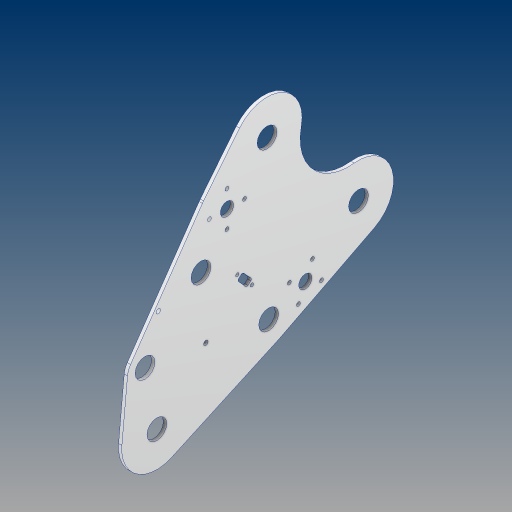
# Autodesk Inventor part: SHOT_1_001_ShooterPlate
Saved by Autodesk Inventor 2024.3 (Build 283343000, 343)
## iProperties
Created: 2024-08-07
Part Number: SHOT_1_001_ShooterPlate
Material: Aluminum 6061
Document SubType Name: Modeling
Designer: Kenji
Density: 2.7 g/cm^3
Appearance: Aluminum - Flat
Mass: 320.131 g
Surface Area: 825.953 cm^2
Volume: 118.567 cm^3
Author: Kenji
Autodesk Inventor part; units mm, degrees
ref_plane "YZ Plane" through (0, 0, 0) normal (1, 0, 0) x (0, 1, 0)
ref_plane "XZ Plane" through (0, 0, 0) normal (0, 1, 0) x (-1, 0, 0)
ref_plane "XY Plane" through (0, 0, 0) normal (0, 0, 1) x (1, 0, 0)
sketch "Sketch1" plane through (0, 0, 0) normal (1, 0, 0) x (0, 1, 0)
  line L0 (0, 0) -> (355.6, 0) construction
  line L1 (0, -355.6) -> (0, 0) construction
  line L2 (0, -292.1) -> (279.4, -292.1) construction
  circle A0 centre (336.7111, -261.0807) radius 50.8 construction
  circle A1 centre (191.0749, -393.5194) radius 50.8 construction
  circle A2 centre (263.893, -327.3) radius 50.8 construction
  circle A3 centre (191.0749, -393.5194) radius 47.625 construction
  circle A4 centre (336.7111, -261.0807) radius 47.625 construction
  line L3 (336.7111, -261.0807) -> (191.0749, -393.5194) construction
  circle A5 centre (336.7111, -261.0807) radius 14.2875
  circle A6 centre (191.0749, -393.5194) radius 14.2875
  circle A7 centre (215.3861, -165.4189) radius 25.4 construction
  circle A8 centre (107.6199, -263.4194) radius 25.4 construction
  circle A9 centre (107.6199, -263.4194) radius 22.225 construction
  circle A10 centre (215.3861, -165.4189) radius 22.225 construction
  circle A11 centre (215.3861, -165.4189) radius 14.2875
  circle A12 centre (107.6199, -263.4194) radius 14.2875
  line L4 (301.4765, -293.1223) -> (198.9433, -180.3717) construction
  line L5 (226.3095, -361.4778) -> (123.7762, -248.7272) construction
  circle A13 centre (161.3598, -214.5495) radius 50.8 construction
  line L6 (215.3861, -165.4189) -> (107.6199, -263.4194) construction
  circle A14 centre (50.8, -101.6) radius 50.8 construction
  circle A15 centre (25.4, -170.0653) radius 25.4 construction
  circle A16 centre (25.4, -170.0653) radius 22.225 construction
  circle A17 centre (25.4, -170.0653) radius 14.2875 construction
  circle A18 centre (136.3874, -84.4507) radius 25.4 construction
  circle A19 centre (136.3874, -84.4507) radius 22.225 construction
  circle A20 centre (136.3874, -84.4507) radius 14.2875
  circle A21 centre (50.8, -101.6) radius 14.2875
  circle A22 centre (41.2055, -25.7462) radius 25.4 construction
  circle A23 centre (41.2055, -25.7462) radius 22.225 construction
  circle A24 centre (41.2055, -25.7462) radius 14.2875 construction
  circle A25 centre (-111.1945, -98.7712) radius 50.8 construction
  circle A26 centre (41.2055, -98.7712) radius 50.8 construction
  line L7 (-111.1945, -47.9712) -> (41.2055, -47.9712) construction
  line L8 (-111.1945, -149.5712) -> (41.2055, -149.5712) construction
  circle A27 centre (276.2209, -203.0571) radius 30 construction
  circle A28 centre (276.2209, -203.0571) radius 25.4 construction
  circle A29 centre (301.6209, -203.0571) radius 2.794
  circle A30 centre (294.1814, -185.0966) radius 2.794
  circle A31 centre (276.2209, -177.6571) radius 2.794
  circle A32 centre (258.2604, -185.0966) radius 2.794
  circle A33 centre (250.8209, -203.0571) radius 2.794
  circle A34 centre (258.2604, -221.0176) radius 2.794
  circle A35 centre (276.2209, -228.4571) radius 2.794
  circle A36 centre (294.1814, -221.0176) radius 2.794
  circle A37 centre (276.2209, -203.0571) radius 9.652
  line L9 (250.7089, -187.273) -> (236.9862, -178.7828) construction
  circle A38 centre (276.2209, -203.0571) radius 9.5504 construction
  circle A39 centre (336.7111, -261.0807) radius 9.5504 construction
  circle A40 centre (336.7111, -261.0807) radius 14.3256 construction
  circle A41 centre (215.3861, -165.4189) radius 14.3256 construction
  circle A42 centre (136.3874, -84.4507) radius 14.3256 construction
  circle A43 centre (215.3861, -165.4189) radius 14.3256 construction
  circle A44 centre (123.5241, -172.549) radius 6.35 construction
  circle A45 centre (123.5241, -172.549) radius 3.2512
  line L10 (122.4294, -178.8039) -> (111.9989, -238.3998) construction
  arc A46 (325.875, -310.7115) -> (241.5089, -387.4324) centre (310.9542, -379.0508) ccw
  arc A47 (325.875, -310.7115) -> (368.3984, -221.3748) centre (336.7111, -261.0807) ccw
  arc A48 (145.82, -416.5983) -> (241.5089, -387.4324) centre (191.0749, -393.5194) ccw
  line L11 (138.8602, -59.1713) -> (55.7455, -51.0413)
  arc A49 (150.8617, -63.5783) -> (138.8602, -59.1713) centre (136.3874, -84.4507) ccw
  arc A50 (55.7455, -51.0413) -> (4.5541, -122.6227) centre (50.8, -101.6) ccw
  circle A51 centre (197.6195, -103.7307) radius 6.35 construction
  circle A52 centre (197.6195, -103.7307) radius 3.2512
  line L12 (161.503, -214.4192) -> (263.893, -327.3) construction
  circle A53 centre (128.5074, -316.6157) radius 30 construction
  circle A54 centre (128.5074, -316.6157) radius 25.4 construction
  circle A55 centre (152.1501, -307.3324) radius 2.794 construction
  line L13 (191.5627, -101.8236) -> (160.6148, -92.0791) construction
  line L14 (199.3769, -109.8327) -> (208.3565, -141.0111) construction
  line L15 (116.9032, -287.0622) -> (117.5428, -288.6911) construction
  circle A56 centre (128.5074, -316.6157) radius 22.86 construction
  circle A57 centre (107.6199, -263.4194) radius 34.29 construction
  circle A58 centre (138.661, -293.3334) radius 2.794
  circle A59 centre (119.224, -292.9729) radius 2.794 construction
  circle A60 centre (105.2251, -306.462) radius 2.794
  circle A61 centre (104.8646, -325.899) radius 2.794 construction
  circle A62 centre (118.3537, -339.8979) radius 2.794
  circle A63 centre (137.7907, -340.2584) radius 2.794 construction
  circle A64 centre (151.7896, -326.7693) radius 2.794
  line L16 (176.8412, -219.7225) -> (165.2898, -230.2004)
  line L17 (165.1271, -233.5371) -> (168.7791, -237.5632)
  line L18 (172.1157, -237.7258) -> (183.6672, -227.2479)
  line L19 (183.8298, -223.9112) -> (180.1779, -219.8851)
  arc A65 (183.6672, -227.2479) -> (183.8298, -223.9112) centre (182.0802, -225.4982) ccw
  arc A66 (180.1779, -219.8851) -> (176.8412, -219.7225) centre (178.4283, -221.4722) ccw
  arc A67 (168.7791, -237.5632) -> (172.1157, -237.7258) centre (170.5287, -235.9761) ccw
  arc A68 (165.2898, -230.2004) -> (165.1271, -233.5371) centre (166.8768, -231.9501) ccw
  line L20 (186.1428, -218.1438) -> (162.8049, -239.3128) construction
  circle A69 centre (186.1428, -218.1438) radius 2.3876
  circle A70 centre (162.8049, -239.3128) radius 2.3812
  circle A71 centre (128.5074, -316.6157) radius 9.5504
  circle A72 centre (276.2209, -203.0571) radius 30.48 construction
  circle A73 centre (336.7111, -261.0807) radius 41.91 construction
  circle A74 centre (276.2209, -203.0571) radius 41.91 construction
  circle A75 centre (128.5074, -316.6157) radius 19.1008 construction
  circle A76 centre (215.3861, -165.4189) radius 19.1008 construction
  circle A77 centre (136.3874, -84.4507) radius 19.1008 construction
  circle A78 centre (276.2209, -203.0571) radius 19.1008 construction
  circle A79 centre (191.0749, -393.5194) radius 19.1008 construction
  line L21 (4.5541, -122.6227) -> (75.2478, -278.1353)
  line L22 (75.9415, -279.5746) -> (145.82, -416.5983)
  arc A80 (75.2478, -278.1353) -> (75.9415, -279.5746) centre (107.6199, -263.4194) ccw
  circle A81 centre (276.2209, -203.0571) radius 43.18 construction
  line L23 (303.1551, -169.3072) -> (368.3984, -221.3748)
  line L24 (150.8617, -63.5783) -> (300.8271, -167.5741)
  arc A82 (303.1551, -169.3072) -> (300.8271, -167.5741) centre (276.2209, -203.0571) ccw
  circle A83 centre (107.6199, -263.4194) radius 35.56 construction
  point P0 (33.8339, -53.7169)
  point P1 (178.5909, -218.1355)
  point P2 (163.5401, -231.7874)
  point P3 (170.3661, -239.3128)
  point P4 (171.0655, -224.9614)
  point P5 (182.0039, -221.8981)
  point P6 (182.0039, -221.8981)
  dimension "d44" = 101.6
  dimension "d81" = 60
  dimension "d82" = 50.8
  dimension "d102" = 12.7
  dimension "d268" = 60
  dimension "d269" = 50.8
  dimension "d13" = 355.6
  dimension "d14" = 355.6
  dimension "d15" = 292.1
  dimension "d29" = 101.6
  dimension "d31" = 3.175
  dimension "d36" = 28.575
  dimension "d38" = 50.8
  dimension "d39" = 3.175
  dimension "d41" = 28.575
  dimension "d42" = 152.4
  dimension "d43" = 152.4
  dimension "d46" = 279.4
  dimension "d47" = 101.6
  dimension "d50" = 101.6
  dimension "d51" = 145.6628
  dimension "d60" = 28.575
  dimension "d61" = 113.1223
  dimension "d77" = 101.6
  dimension "d78" = 101.6
  dimension "d79" = 152.4
  dimension "d80" = 41.2055
  dimension "d83" = 5.588
  dimension "d86" = 360
  dimension "d88" = 19.304
  dimension "d91" = 19.1008
  dimension "d92" = 19.1008
  dimension "d93" = 28.6512
  dimension "d94" = 28.6512
  dimension "d95" = 28.6512
  dimension "d96" = 28.6512
  dimension "d103" = 6.5024
  dimension "d108" = 12.7
  dimension "d109" = 6.5024
  dimension "d114" = 101.6
  dimension "d116" = 87.2886
  dimension "d117" = 158.0611
  dimension "d119" = 323.8734
  dimension "d121" = 42.21
  dimension "d270" = 5.588
  dimension "d279" = 45.72
  dimension "d280" = 68.58
  dimension "d283" = 360
  dimension "d285" = 20.32
  dimension "d286" = 10.16
  dimension "d287" = 10.16
  dimension "d288" = 2.3622
  dimension "d289" = 2.3622
  dimension "d291" = 5.08
  dimension "d292" = 4.7752
  dimension "d293" = 4.7625
  dimension "d294" = 5.6005
  dimension "d295" = 5.588
  dimension "d296" = 19.1008
  dimension "d297" = 60.96
  dimension "d300" = 83.82
  dimension "d301" = 83.82
  dimension "d302" = 38.2016
  dimension "d303" = 38.2016
  dimension "d304" = 38.2016
  dimension "d305" = 38.2016
  dimension "d306" = 38.2016
  dimension "d309" = 1.27
  dimension "d312" = 1.27
  dimension "d314" = 208.6282
  constraints: 76 centre point, 50 end point, 46 point on circle, 37 tangent, 32 coincident, 22 point on line, 18 equal radius, 6 midpoint, 5 concentric, 5 perpendicular, 3 horizontal, 2 horizontal alignment, 2 parallel, 1 equal length, 1 vertical alignment, 67 other
  measures "d13" distance of L1.start L0.start
  measures "d14" distance of L0.start L0.end
  measures "d15" distance between parallel lines of L0 L2
  measures "d29" diameter of A1
  measures "d31" radial gap between concentric circles of A1 A3
  measures "d36" diameter of A5
  measures "d38" diameter of A8
  measures "d39" radial gap between concentric circles of A8 A9
  measures "d41" diameter of A12
  measures "d42" distance of L4.start L4.end
  measures "d43" distance of L5.start L5.end
  measures "d46" distance of L2.start L2.end
  measures "d47" diameter of A14
  measures "d50" distance from line of L0 A14.centre
  measures "d51" distance of L6.start L6.end
  measures "d60" diameter of A21
  measures "d61" distance of A19.centre A7.centre
  measures "d77" diameter of A25
  measures "d78" diameter of A26
  measures "d79" distance of L8.start L8.end
  measures "d80" distance from line of L1 A22.centre
  measures "d83" diameter of A29
  measures "d88" diameter of A37
  measures "d91" diameter of A38
  measures "d92" diameter of A39
  measures "d93" diameter of A40
  measures "d94" diameter of A41
  measures "d95" diameter of A42
  measures "d96" diameter of A43
  measures "d103" diameter of A45
  measures "d108" diameter of A51
  measures "d109" diameter of A52
  measures "d114" distance of point (123.524, -172.549) A14.centre
  measures "d116" distance of A14.centre A19.centre
  measures "d117" distance of A14.centre L12.start
  measures "d119" distance of A14.centre L3.end
  measures "d121" angle of L1 L12
  measures "d270" diameter of A55
  measures "d279" diameter of A56
  measures "d280" diameter of A57
  measures "d285" distance of point (178.591, -218.135) point (163.54, -231.787)
  measures "d286" distance of point (163.54, -231.787) point (170.366, -239.313)
  measures "d287" distance of point (178.591, -218.135) point (171.065, -224.961)
  measures "d288" radius of A65
  measures "d289" radius of A67
  measures "d291" distance between parallel lines of L16 L20
  measures "d292" diameter of A69
  measures "d293" diameter of A70
  measures "d294" distance from line of L17 L20.end
  measures "d295" distance from line of L19 A69.centre
  measures "d296" diameter of A71
  measures "d297" diameter of A72
  measures "d300" diameter of A73
  measures "d301" diameter of A74
  measures "d302" diameter of A75
  measures "d303" diameter of A76
  measures "d304" diameter of A77
  measures "d305" diameter of A78
  measures "d306" diameter of A79
  measures "d309" radial gap between concentric circles of A74 A81
  measures "d314" distance of L3.end point (276.221, -203.057)
extrude "Extrusion6" add sketch "Sketch1" along normal blind 4.7625 contours A30 | A32 | A34 | A36 | A46 A48 L22 A80 L21 A50 L11 A49 L24 A82 L23 A47
body "Solid3"
